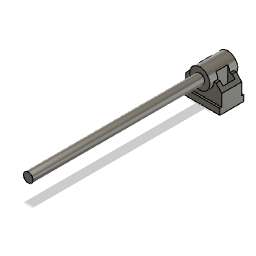
Detail_rode v1 (Autodesk Fusion 360 design; units mm, degrees)
Autodesk Fusion 360 part; units mm, degrees
sketch "Sketch1" plane through (0, 0, 0) normal (0, 1, 0) x (1, 0, 0)
  line L0 (45, -30) -> (-45, -30)
  line L1 (-45, -30) -> (-45, 30)
  line L2 (-45, 30) -> (45, 30)
  line L3 (45, 30) -> (45, -30)
  line L4 (45, -30) -> (-45, 30) construction
  line L5 (-45, -30) -> (45, 30) construction
  dimension "d1" = 90
  dimension "d2" = 60
  constraint horizontal L0
  constraint perpendicular L0 L1
  constraint parallel L0 L2
  constraint parallel L1 L3
  constraint coincident L4 origin
  constraint coincident L5 origin
  measures "d1" distance of L1.end L2.end
  measures "d2" distance of L0.end L1.end
extrude "Extrude1" add sketch "Sketch1" along normal blind 15 makes body 1
sketch "Sketch2" plane through (0, 0, 30) normal (0, 0, 1) x (1, 0, 0)
  line L0 (-45, 0) -> (45, 0)
  line L1 (45, 0) -> (45, 15)
  line L2 (45, 15) -> (-45, 15)
  line L3 (-45, 15) -> (-45, 0)
  line L4 (-45, 15) -> (-45, 45)
  line L5 (45, 15) -> (45, 45)
  line L6 (0, 15) -> (0, 60) construction
  arc A0 (-25, 60) -> (25, 60) centre (0, 60) ccw
  line L7 (-45, 45) -> (-31, 45) construction
  line L8 (45, 45) -> (31, 45) construction
  line L9 (-31, 45) -> (-31, 60) construction
  line L10 (31, 45) -> (31, 60) construction
  line L11 (-45, 45) -> (-31, 60)
  line L12 (-31, 60) -> (-25, 60)
  line L13 (25, 60) -> (31, 60)
  line L14 (31, 60) -> (45, 45)
  dimension "d5" = 30
  dimension "d6" = 45
  dimension "d7" = 25
  dimension "d8" = 14
  dimension "d9" = 14
  dimension "d10" = 15
  dimension "d11" = 15
  constraint coincident L2.end L3.start
  constraint perpendicular L2 L4
  constraint coincident L1.end L2.start
  constraint perpendicular L2 L5
  constraint equal L4 L5
  constraint midpoint L2 L6.start
  constraint perpendicular L2 L6
  constraint coincident L6.end A0.centre
  constraint perpendicular L4 L7
  constraint perpendicular L5 L8
  constraint perpendicular L7 L9
  constraint perpendicular L8 L10
  constraint perpendicular L9 L12
  constraint perpendicular L10 L13
  measures "d5" distance of L2.end L4.end
  measures "d6" distance of L6.start L6.end
  measures "d7" radius of A0
  measures "d8" distance of L4.end L7.end
  measures "d9" distance of L5.end L8.end
  measures "d10" distance of L7.end L9.end
  measures "d11" distance of L8.end L10.end
extrude "Extrude2" add sketch "Sketch2" along normal blind -5 and the other way blind 55 contours L2 L4 L5 A0 L11 L12 L13 L14 bodies 1
sketch "Sketch3" plane through (0, 0, 25) normal (0, 0, 1) x (1, 0, 0)
  line L0 (45, 15) -> (45, 45)
  line L1 (45, 45) -> (31, 60)
  line L2 (31, 60) -> (25, 60)
  arc A0 (-25, 60) -> (25, 60) centre (0, 60) ccw
  line L3 (-25, 60) -> (-31, 60)
  line L4 (-31, 60) -> (-45, 45)
  line L5 (-45, 45) -> (-45, 15)
  line L6 (-45, 15) -> (45, 15)
  circle A1 centre (0, 60) radius 25
  circle A2 centre (0, 60) radius 12
  dimension "d16" = 50
  dimension "d17" = 24
  constraint concentric A0 A1
  constraint concentric A1 A2
  measures "d16" diameter of A1
  measures "d17" diameter of A2
extrude "Extrude3" add sketch "Sketch3" along normal blind 10 and the other way blind 60 contours A0 A1 bodies 1
sketch "Sketch4" plane through (0, 60, 0) normal (0, 1, 0) x (-1, 0, 0)
  line L0 (31, 25) -> (25, 25)
  line L1 (25, 25) -> (25, -25)
  line L2 (25, -25) -> (31, -25)
  line L3 (31, -25) -> (31, 25)
  line L4 (38, -15) -> (20, -15)
  line L5 (20, -15) -> (20, 15)
  line L6 (20, 15) -> (38, 15)
  line L7 (38, 15) -> (38, -15)
  line L8 (45, 25) -> (45, -25)
  line L9 (45, -25) -> (31, -25)
  line L10 (-20, 15) -> (-20, -15)
  line L11 (-20, -15) -> (-38, -15)
  line L12 (-38, -15) -> (-38, 15)
  line L13 (-38, 15) -> (-20, 15)
  dimension "d22" = 18
  dimension "d23" = 30
  dimension "d24" = 7
  dimension "d25" = 10
  dimension "d28" = -58
  dimension "d29" = 0
  dimension "d30" = 40
  constraint horizontal L4
  constraint vertical L5
  constraint horizontal L6
  constraint vertical L7
  measures "d22" distance of L4.start L4.end
  measures "d23" distance of L4.start L6.end
  measures "d24" distance of L7 L8
  measures "d25" distance of L4 L9
  measures "d30" distance of L5 L10
extrude "Extrude4" cut sketch "Sketch4" along normal blind 50 and the other way blind 60 contours L3 L4 L6 L7 | L1 L3 L4 L6 | L1 L4 L5 L6 | L10 L11 L12 L13 bodies 1
sketch "Sketch5" plane through (0, 0, 35) normal (0, 0, 1) x (1, 0, 0)
  circle A0 centre (0, 60) radius 12
  circle A1 centre (0, 60) radius 25
  circle A2 centre (0, 60) radius 12
  dimension "d35" = 24
  constraint concentric A0 A2
  measures "d35" diameter of A2
extrude "Extrude5" add sketch "Sketch5" along normal blind 430 and the other way blind 70 separate body contours A0 A2 makes body 2
copy_body "Body->Comp1" bodies 1 removing the originals makes body 3 in component "Detail"
copy_body "Body->Comp2" bodies 2 removing the originals makes body 4 in component "Rod"
component "Detail" placed x (1, 0, 0) y (0, 1, 0) z (0, 0, 1) at (0, 0, 0)
component "Rod" placed x (1, 0, 0) y (0, 1, 0) z (0, 0, 1) at (0, 0, 0)
